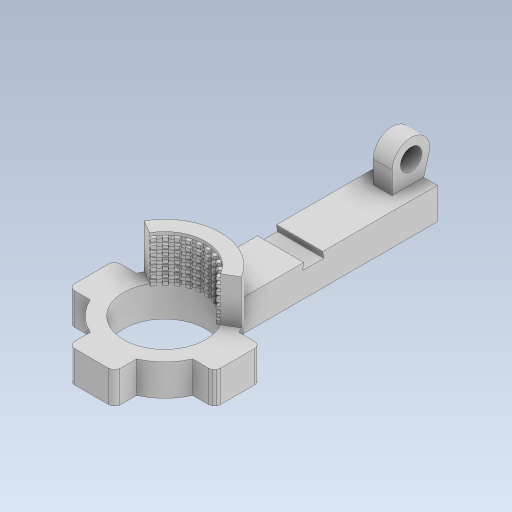
# Autodesk Inventor part: Slider2
Saved by Autodesk Inventor 2023 (Build 270158000, 158)
## iProperties
Created: 2022-09-14
Part Number: Slider2
Material: Generic
Document SubType Name: Modeling
Designer: Dave
Density: 1 g/cm^3
Appearance: Default
Author: Dave
Autodesk Inventor part; units mm, degrees
ref_plane "YZ Plane" through (0, 0, 0) normal (1, 0, 0) x (0, 1, 0)
ref_plane "XZ Plane" through (0, 0, 0) normal (0, 1, 0) x (-1, 0, 0)
ref_plane "XY Plane" through (0, 0, 0) normal (0, 0, 1) x (1, 0, 0)
sketch "Sketch1" plane through (0, 0, 0) normal (0, 1, 0) x (-1, 0, 0)
  arc A0 (16.223, 7.3) -> (7.325, 16.198) centre (0, -0.025) ccw
  line L0 (7.325, 16.198) -> (7.325, 21.125)
  arc A1 (7.325, 21.125) -> (7.025, 22.1786) centre (5.325, 21.125) ccw
  arc A2 (7.025, 22.1786) -> (6.3786, 22.825) centre (5.325, 21.125) ccw
  arc A3 (6.3786, 22.825) -> (5.325, 23.125) centre (5.325, 21.125) ccw
  line L1 (5.325, 23.125) -> (-5.325, 23.125)
  arc A4 (-5.325, 23.125) -> (-6.3786, 22.825) centre (-5.325, 21.125) ccw
  arc A5 (-6.3786, 22.825) -> (-7.025, 22.1786) centre (-5.325, 21.125) ccw
  arc A6 (-7.025, 22.1786) -> (-7.325, 21.125) centre (-5.325, 21.125) ccw
  line L2 (-7.325, 21.125) -> (-7.325, 16.198)
  arc A7 (-7.325, 16.198) -> (-16.223, 7.3) centre (0, -0.025) ccw
  line L3 (-16.223, 7.3) -> (-21.1473, 7.3)
  ellipse E0 centre (-21.2521, 5.3) end of major axis (-19.7618, 6.7142) minor radius 1.9496 (-21.1473, 7.3) -> (-22.218, 7) ccw
  ellipse E1 centre (-21.163, 5.3) end of major axis (-23.1657, 5.3) minor radius 2 (-22.218, 7) -> (-22.85, 6.3778) ccw
  ellipse E2 centre (-21.247, 5.3) end of major axis (-21.247, 7.3) minor radius 1.903 (-22.85, 6.3778) -> (-23.15, 5.3) ccw
  line L4 (-23.15, 5.3) -> (-23.15, -5.35)
  ellipse E3 centre (-21.247, -5.35) end of major axis (-21.247, -3.35) minor radius 1.903 (-23.15, -5.35) -> (-22.85, -6.4278) ccw
  ellipse E4 centre (-21.163, -5.35) end of major axis (-23.1657, -5.35) minor radius 2 (-22.85, -6.4278) -> (-22.218, -7.05) ccw
  ellipse E5 centre (-21.2521, -5.35) end of major axis (-22.7423, -3.9358) minor radius 1.9496 (-22.218, -7.05) -> (-21.1473, -7.35) ccw
  line L5 (-21.1473, -7.35) -> (-16.223, -7.35)
  arc A8 (-16.223, -7.35) -> (-7.325, -16.248) centre (0, -0.025) ccw
  line L6 (-7.325, -16.248) -> (-7.325, -21.175)
  line L7 (-7.025, -22.2286) -> (-7.025, -16.0531)
  arc A9 (-7.325, -21.175) -> (-7.025, -22.2286) centre (-5.325, -21.175) ccw
  arc A10 (-7.025, -22.2286) -> (-6.3786, -22.875) centre (-5.325, -21.175) ccw
  arc A11 (-6.3786, -22.875) -> (-5.325, -23.175) centre (-5.325, -21.175) ccw
  line L8 (-5.325, -23.175) -> (5.325, -23.175)
  line L9 (7.325, -21.175) -> (7.325, -16.248)
  arc A12 (7.025, -22.2286) -> (7.325, -21.175) centre (5.325, -21.175) ccw
  arc A13 (6.3786, -22.875) -> (7.025, -22.2286) centre (5.325, -21.175) ccw
  arc A14 (5.325, -23.175) -> (6.3786, -22.875) centre (5.325, -21.175) ccw
  arc A15 (7.325, -16.248) -> (16.223, -7.35) centre (0, -0.025) ccw
  line L10 (16.223, -7.35) -> (21.1473, -7.35)
  ellipse E6 centre (21.2521, -5.35) end of major axis (19.7618, -6.7642) minor radius 1.9496 (21.1473, -7.35) -> (22.218, -7.05) ccw
  ellipse E7 centre (21.163, -5.35) end of major axis (23.1657, -5.35) minor radius 2 (22.218, -7.05) -> (22.85, -6.4278) ccw
  ellipse E8 centre (21.247, -5.35) end of major axis (21.247, -7.35) minor radius 1.903 (22.85, -6.4278) -> (23.15, -5.35) ccw
  line L11 (23.15, -5.35) -> (23.15, 5.3)
  ellipse E9 centre (21.247, 5.3) end of major axis (21.247, 3.3) minor radius 1.903 (23.15, 5.3) -> (22.85, 6.3778) ccw
  ellipse E10 centre (21.163, 5.3) end of major axis (23.1657, 5.3) minor radius 2 (22.85, 6.3778) -> (22.218, 7) ccw
  ellipse E11 centre (21.2521, 5.3) end of major axis (22.7423, 3.8858) minor radius 1.9496 (22.218, 7) -> (21.1473, 7.3) ccw
  line L12 (21.1473, 7.3) -> (16.223, 7.3)
  circle A16 centre (0, -0.025) radius 13
  point P0 (0, 0)
  point P1 (0, 0)
  dimension "d0" = 26
  constraints: 32 point on circle, 26 end point, 17 centre point, 1 coincident, 1 vertical, 49 other
  measures "d0" diameter of A16
extrude "Extrusion1" add sketch "Sketch1" along normal blind 10
sketch "Sketch2" plane through (0, 10, 0) normal (0, 1, 0) x (1, 0, 0)
  circle A0 centre (0, 0.025) radius 13 projected
  line L0 (-13, 0.025) -> (-17.8, 0.025)
  arc A1 (17.8, 0.025) -> (-17.8, 0.025) centre (0, 0.025) ccw
  arc A2 (-7.325, 16.248) -> (-16.223, 7.35) centre (0, 0.025) ccw projected
  line L1 (13, 0.025) -> (17.8, 0.025)
  line L2 (-15.4153, 8.925) -> (-10.3923, 6.025)
  line L3 (10.3923, 6.025) -> (15.4153, 8.925)
  arc A3 (16.223, 7.35) -> (7.325, 16.248) centre (0, 0.025) ccw projected
  line L4 (0, 32.435) -> (0, -32.385) projected
  circle A4 centre (0, 0.025) radius 12
  point P0 (0, 0)
  point P1 (-11.2583, 6.525)
  point P2 (11.2583, 6.525)
  dimension "d3" = 120
  dimension "d6" = 1
  constraints: 10 point on circle, 8 end point, 2 centre point, 2 coincident, 2 horizontal, 2 horizontal alignment, 2 point on line, 1 concentric, 1 line through centre, 1 other
  measures "d3" angle of L3 L2
  measures "d6" radial gap between concentric circles of A0 A4
extrude "Extrusion2" add sketch "Sketch2" along normal blind 14 contours L3 A4 L4 A0 | A0 L4 A1 L3 | L4 A4 L2 A0 | A0 L2 A1 L4 picked at (10.4372, 7.0912) picked at (-10.4372, 7.0912)
sketch "Sketch3" plane through (0, 24, 0) normal (0, 1, 0) x (1, 0, 0)
  arc A0 (10.3923, 6.025) -> (-10.3923, 6.025) centre (0, 0.025) ccw projected
  circle A1 centre (0, 0) radius 12.0125
  line L0 (-11.2583, 6.525) -> (-10.3923, 6.025) projected
  circle A2 centre (0, 0) radius 13.0125
  line L1 (-10.3923, 6.025) -> (-11.2583, 6.525)
  arc A3 (11.2583, 6.525) -> (-11.2583, 6.525) centre (0, 0.025) ccw projected
  line L2 (-9.6664, 7.1317) -> (-10.4722, 7.7239)
  line L3 (-8.8232, 8.1518) -> (-9.5589, 8.8291)
  line L4 (-7.8729, 9.0729) -> (-8.5297, 9.827)
  line L5 (-6.827, 9.8839) -> (-7.3968, 10.7057)
  line L6 (-5.6983, 10.575) -> (-6.1742, 11.4545)
  line L7 (-4.5004, 11.1377) -> (-4.8767, 12.0642)
  line L8 (-3.2478, 11.5651) -> (-3.5199, 12.5274)
  line L9 (-1.9558, 11.8522) -> (-2.1204, 12.8386)
  line L10 (-0.6401, 11.9955) -> (-0.6952, 12.9939)
  line L11 (0.6834, 11.9931) -> (0.7384, 12.9915)
  line L12 (1.9985, 11.8451) -> (2.1631, 12.8315)
  line L13 (3.2895, 11.5534) -> (3.5616, 12.5156)
  line L14 (4.5405, 11.1214) -> (4.9168, 12.0479)
  line L15 (5.7364, 10.5544) -> (6.2123, 11.4338)
  line L16 (6.8626, 9.8593) -> (7.4324, 10.681)
  line L17 (7.9056, 9.0445) -> (8.5623, 9.7986)
  line L18 (8.8525, 8.1199) -> (9.5883, 8.7972)
  line L19 (9.6921, 7.0968) -> (10.4978, 7.689)
  line L20 (10.414, 5.9875) -> (11.28, 6.4875)
  point P0 (0.0028, 0.0248)
  point P1 (0.0055, 0.0244)
  point P2 (0.0081, 0.0236)
  point P3 (0.0107, 0.0226)
  point P4 (0.0131, 0.0213)
  point P5 (0.0154, 0.0197)
  point P6 (0.0174, 0.0179)
  point P7 (0.0193, 0.0159)
  point P8 (0.0209, 0.0137)
  point P9 (0.0223, 0.0113)
  point P10 (0.0234, 0.0088)
  point P11 (0.0242, 0.0061)
  point P12 (0.0248, 0.0034)
  point P13 (0.025, 0.0007)
  point P14 (0.0249, -0.0021)
  point P15 (0.0245, -0.0048)
  point P16 (0.0239, -0.0075)
  point P17 (0.0229, -0.01)
  point P18 (0.0217, -0.0125)
  point P19 (9.6939, 7.0981)
  point P20 (8.8558, 8.1229)
  point P21 (7.9097, 9.0492)
  point P22 (6.8672, 9.8658)
  point P23 (5.7409, 10.5627)
  point P24 (4.5445, 11.1312)
  point P25 (3.2926, 11.5644)
  point P26 (2.0005, 11.8571)
  point P27 (0.684, 12.0055)
  point P28 (-0.6408, 12.0079)
  point P29 (-1.9578, 11.8642)
  point P30 (-3.251, 11.5762)
  point P31 (-4.5044, 11.1475)
  point P32 (-5.7028, 10.5833)
  point P33 (-6.8316, 9.8906)
  point P34 (-7.8771, 9.0777)
  point P35 (-8.8265, 8.1548)
  point P36 (-9.6683, 7.133)
  dimension "d9" = 120
  constraints: 40 end point, 3 point on circle, 2 coincident, 1 centre point, 80 other
extrude "Extrusion3" cut sketch "Sketch3" against normal up to surface (14 mm away) contours A0 L18 A2 L19 | A0 L16 A2 L17 | L2 A2 L3 A0 | A0 L14 A2 L15 | L4 A2 L5 A0 | A0 L12 A2 L13 | L6 A2 L7 A0 | A0 L10 A2 L11 | L8 A2 L9 A0
sketch "Sketch4" plane through (15.4153, 10, -8.925) normal (0.5, 0, 0.8660254) x (0.8660254, 0, -0.5)
  line L0 (-5.8, 14) -> (0, 14) projected
  line L1 (-5.8, 14) -> (-4.8, 14)
  line L2 (-5.8, 0) -> (-4.8, 0) projected
  line L3 (-5.8, 14) -> (-5.8, 0)
  line L4 (-5.8, 0) -> (-4.8, 0)
  line L5 (-5.498, 14) -> (-5.498, 0) projected
  line L6 (-4.8, 0) -> (-4.8, 14)
  line L7 (-5.8, 13) -> (-4.8, 13)
  line L8 (-5.8, 12) -> (-4.8, 12)
  line L9 (-5.8, 11) -> (-4.8, 11)
  line L10 (-5.8, 10) -> (-4.8, 10)
  line L11 (-5.8, 9) -> (-4.8, 9)
  line L12 (-5.8, 8) -> (-4.8, 8)
  line L13 (-5.8, 7) -> (-4.8, 7)
  line L14 (-5.8, 6) -> (-4.8, 6)
  line L15 (-5.8, 5) -> (-4.8, 5)
  line L16 (-17.8125, -14.8) -> (-17.8125, 18.8) projected
  line L17 (-7.5305, 14) -> (-6.7156, 14) projected
  line L18 (-5.8, 0) -> (-6.7852, 0)
  line L19 (-6.7852, 0) -> (-6.7852, 14)
  line L20 (-6.7852, 14) -> (-5.8, 14)
  line L21 (-5.8, 14) -> (-5.8, 0)
  line L22 (-5.8, 4) -> (-4.8, 4)
  line L23 (-5.8, 3) -> (-4.8, 3)
  line L24 (-5.8, 2) -> (-4.8, 2)
  line L25 (-5.8, 1) -> (-4.8, 1)
  point P0 (-17.8125, -10)
  point P1 (-5.8, 6)
  point P2 (-5.8, 5)
  point P3 (-5.8, 8)
  point P4 (-5.8, 7)
  point P5 (-5.8, 10)
  point P6 (-5.8, 9)
  point P7 (-5.498, 4)
  point P8 (-5.8, 2)
  point P9 (-5.8, 1)
  point P10 (-5.498, 3)
  point P11 (-5.498, 4)
  point P12 (-5.8, 3)
  point P13 (-5.8, 4)
  dimension "d16" = 1
  constraints: 42 end point, 3 equal length, 3 vertical, 2 horizontal, 1 perpendicular, 1 point on line, 39 other
  measures "d16" distance of L0.start L7.start
revolve "Revolution1" cut sketch "Sketch4" angle 360 about axis through (-0.0108, -10, -0.0188) along (0, -1, 0) contours L0 L5 L7 L3 | L3 L18 L19 L17 L20 | L0 L6 L7 L5 | L8 L5 L9 L3 | L8 L6 L9 L5 | L10 L5 L11 L3 | L10 L6 L11 L5 | L3 L24 L5 L25 | L12 L5 L13 L3 | L5 L24 L6 L25 | L12 L6 L13 L5 | L3 L22 L5 L23 | L14 L5 L15 L3 | L5 L22 L6 L23 | L14 L6 L15 L5
sketch "Sketch5" plane through (-5.325, 0, 23.125) normal (0, 0, 1) x (1, 0, 0)
  line L0 (21.548, 0) -> (12.65, 0) projected
  line L1 (-2, 10) -> (12.65, 10)
  line L2 (12.65, 10) -> (12.65, 0)
  line L3 (12.65, 0) -> (-2, 0)
  line L4 (-2, 0) -> (-2, 10)
  point P0 (5.325, 0)
  constraints: 8 end point, 2 parallel, 1 horizontal, 1 perpendicular
extrude "Extrusion4" add sketch "Sketch5" along normal blind 58 and the other way blind 5
sketch "Sketch6" plane through (0, 10, 0) normal (0, 1, 0) x (1, 0, 0)
  line L0 (-7.325, -16.198) -> (-7.325, -81.125) projected
  line L1 (-7.325, -36.7772) -> (7.325, -36.7772)
  line L2 (7.325, -36.7772) -> (7.325, -42.7772)
  line L3 (7.325, -42.7772) -> (-7.325, -42.7772)
  line L4 (-7.325, -42.7772) -> (-7.325, -36.7772)
  line L5 (7.325, -81.125) -> (7.325, -16.198) projected
  circle A0 centre (0, 0) radius 17.7772
  point P0 (-7.325, -42.7772)
  dimension "d28" = 35.5544
  dimension "d26" = 6
  dimension "d27" = 36.7772
  constraints: 8 end point, 2 parallel, 1 coincident, 1 collinear, 1 horizontal, 1 perpendicular, 1 point on line, 3 other
  measures "d26" distance of L3.end L1.start
  measures "d27" distance from line of L1 point (0, 0)
extrude "Extrusion5" cut sketch "Sketch6" against normal blind 2 draft 10 contours L1 L2 L3 L0
sketch "Sketch7" plane through (0, 10, 0) normal (0, 1, 0) x (1, 0, 0)
  line L0 (-7.325, -81.125) -> (7.325, -81.125) projected
  line L1 (-3, -81.125) -> (3, -81.125)
  line L2 (3, -81.125) -> (3, -69.125)
  line L3 (3, -69.125) -> (-3, -69.125)
  line L4 (-3, -69.125) -> (-3, -81.125)
  point P0 (0, 0)
  point P1 (0, -81.125)
  dimension "d31" = 6
  dimension "d32" = 12
  constraints: 8 end point, 2 midpoint, 2 parallel, 1 horizontal, 1 perpendicular, 1 point on line
  measures "d31" distance of L3.end L2.end
  measures "d32" distance of L3.end L1.start
extrude "Extrusion6" add sketch "Sketch7" along normal blind 15
sketch "Sketch8" plane through (3, 10, 81.125) normal (1, 0, 0) x (0, 0, -1)
  line L0 (0, 0) -> (38.3478, 0) projected
  line L1 (0, 15) -> (12, 15) projected
  point P0 (81.125, -10)
  point P1 (6, 7)
  point P2 (6, 15)
  dimension "d35" = 7
  constraints: 1 midpoint, 1 vertical alignment
  measures "d35" distance from line of L0 point (6, 7)
hole "Hole1" at (3, 17, 75.125) direction (-1, 0, 0) diameter 6.7564 end through all clearance for "Flat Head Machine Screw (82)" size "1/4" standard "Ansi Unified Screw Threads"
mirror "Mirror1" about plane through (0, 0, 0) normal (0, 0, 1) of "Hole1", "Extrusion6", "Extrusion5", "Extrusion4"
sketch "Sketch9" plane through (0, 10, 0) normal (0, 1, 0) x (1, 0, 0)
  ellipse E0 centre (21.2521, -5.3) end of major axis (19.7618, -6.7142) minor radius 1.9496 (21.1473, -7.3) -> (22.218, -7) ccw projected
  ellipse E1 centre (21.163, -5.3) end of major axis (23.1657, -5.3) minor radius 2 (22.218, -7) -> (22.85, -6.3778) ccw projected
  ellipse E2 centre (21.247, -5.3) end of major axis (21.247, -7.3) minor radius 1.903 (22.85, -6.3778) -> (23.15, -5.3) ccw projected
  ellipse E3 centre (21.247, 5.35) end of major axis (21.247, 3.35) minor radius 1.903 (23.15, 5.35) -> (22.85, 6.4278) ccw projected
  ellipse E4 centre (21.163, 5.35) end of major axis (23.1657, 5.35) minor radius 2 (22.85, 6.4278) -> (22.218, 7.05) ccw projected
  ellipse E5 centre (21.2521, 5.35) end of major axis (22.7423, 3.9358) minor radius 1.9496 (22.218, 7.05) -> (21.1473, 7.35) ccw projected
  line L0 (21.1473, 7.35) -> (16.223, 7.35) projected
  ellipse E6 centre (21.247, -5.3) end of major axis (21.247, -7.3) minor radius 1.903 (22.85, -6.3778) -> (23.15, -5.3) ccw projected
  line L1 (16.223, -7.3) -> (21.15, -7.3)
  line L2 (23.15, -5.3) -> (23.15, 5.35)
  line L3 (21.15, 7.35) -> (16.223, 7.35)
  arc A0 (23.15, 5.35) -> (21.15, 7.35) centre (21.15, 5.35) ccw
  arc A1 (21.15, -7.3) -> (23.15, -5.3) centre (21.15, -5.3) ccw
  line L4 (7.35, -21.15) -> (7.35, -16.223)
  line L5 (-5.3, -23.15) -> (5.35, -23.15)
  arc A2 (5.35, -23.15) -> (7.35, -21.15) centre (5.35, -21.15) ccw
  arc A3 (-7.3, -21.15) -> (-5.3, -23.15) centre (-5.3, -21.15) ccw
  line L6 (-7.3, -16.223) -> (-7.3, -21.15)
  line L7 (-7.3, -21.15) -> (-28.9204, -94.0756)
  line L8 (-28.9204, -94.0756) -> (36.4754, -97.0481)
  line L9 (36.4754, -97.0481) -> (7.325, -21.15)
  line L10 (7.325, -16.198) -> (7.325, -81.125) projected
  point P0 (0, 0)
  point P1 (23.15, 7.35)
  point P2 (7.35, -23.15)
  point P3 (7.349, -21.2125)
  dimension "d43" = 2
  dimension "d46" = 90
  constraints: 18 end point, 8 point on circle, 6 point on line, 4 centre point, 4 tangent, 1 collinear, 1 equal radius, 1 horizontal, 1 perpendicular, 22 other
  measures "d43" radius of A0
extrude "Extrusion7" cut sketch "Sketch9" along normal through all both and the other way through all contours L5 A2 L9 L8 L7 A3
sketch "Sketch10" plane through (7.325, 0, -16.248) normal (1, 0, 0) x (0, 0, -1)
  circle A0 centre (58.877, 17) radius 3.3782 projected
  arc A1 (64.877, 17) -> (63.9714, 13.8302) centre (58.877, 17) ccw
  line L0 (64.877, 10) -> (64.877, 25) projected
  line L1 (64.877, 10) -> (64.877, 25) projected
  line L2 (64.877, 17) -> (64.877, 0)
  line L3 (64.877, 0) -> (62.877, 0)
  line L4 (0, 0) -> (64.877, 0) projected
  line L5 (62.877, 0) -> (62.877, 12.5279)
  line L6 (52.877, 10) -> (64.877, 10) projected
  line L7 (62.877, 10) -> (64.877, 10)
  line L8 (62.877, 10) -> (64.877, 17)
  line L9 (52.877, 10) -> (52.877, 25) projected
  circle A2 centre (58.877, 17) radius 3.3782 projected
  line L10 (64.877, 10) -> (52.877, 10) projected
  line L11 (64.877, 10) -> (64.877, 25) projected
  line L12 (64.877, 25) -> (52.877, 25) projected
  line L13 (52.877, 10) -> (52.877, 25) projected
  point P0 (-16.248, 0)
  point P1 (52.877, 17)
  dimension "d50" = 2
  constraints: 10 end point, 5 point on line, 3 point on circle, 1 centre point, 1 coincident, 1 collinear, 1 perpendicular, 1 tangent
  measures "d50" distance of L2.end L3.end
extrude "Extrusion8" cut sketch "Sketch10" against normal through all contours L8 L0 L6 | L9 L12 L0 A1 | L6 L2 L3 L5
body "Solid1"
